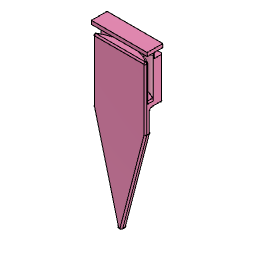
Fliegenfallenkleberfesthalter (Autodesk Fusion 360 design; units mm, degrees)
Autodesk Fusion 360 part; units mm, degrees
note: some values were not read from the file. Set by a fixed rule: which sketch regions a step uses.
sketch "Sketch1" plane through (0, 0, 0) normal (0, 0, 1) x (1, 0, 0)
  line L0 (0, 5) -> (15, 5)
  line L1 (15, 5) -> (15, 0)
  line L2 (15, 0) -> (0, 0)
  line L3 (0, 0) -> (0, 5)
  arc A0 (15, 0.75) -> (0, 0.75) centre (7.5, -11.5062) ccw
  arc A1 (15, 2.25) -> (0, 2.25) centre (7.5, -10.8125) ccw
  line L4 (0, 4.25) -> (15, 4.25) construction
  line L5 (0, 1.5) -> (15, 1.5)
  arc A2 (15, 2.5) -> (0, 2.5) centre (7.5, -10.5625) ccw
  dimension "d1" = 1.5
  dimension "d2" = 1.5
  dimension "d3" = 0.75
  dimension "d4" = 15
  dimension "d5" = 5
  dimension "d9" = 0.75
  dimension "d14" = 1.5
  dimension "d25" = 0.25
  dimension "d26" = 0.25
  constraint horizontal L0
  constraint vertical L1
  constraint horizontal L2
  constraint vertical L3
  constraint coincident L1 A0.start
  constraint coincident L3 A0.end
  constraint tangent A0 A1
  constraint coincident L1 A1.start
  constraint coincident L3 A1.end
  constraint coincident L2.end L3.start
  constraint horizontal A0.end A0.start
  constraint coincident L3 L4.start
  constraint coincident L1 L4.end
  constraint horizontal L4
  constraint tangent A1 L4
  constraint coincident L3 L5.start
  constraint coincident L1 L5.end
  constraint perpendicular L1 L5
  constraint coincident L1 A2.start
  constraint coincident L3 A2.end
  constraint equal A1 A2
  measures "d1" distance of A0.start A1.start
  measures "d2" distance of A0.end A1.end
  measures "d3" distance of L2.end A0.end
  measures "d4" distance of L1.end L2.end
  measures "d5" distance of L0.start L2.end
  measures "d9" distance of L0 L4
  measures "d14" distance of L2 L5
  measures "d25" distance of A1.start A2.start
  measures "d26" distance of A1.end A2.end
extrude "Extrude1" add sketch "Sketch1" against normal blind 2
extrude "Extrude2" add sketch "Sketch1" along normal blind 10 contours L0 L1 L3 A2 | L1 L3 A1 A2 | L1 L2 L3 A0 L5 | A0 L5
extrude "Extrude3" add sketch "Sketch1" against normal blind 35 contours L3 A0 L5 | L1 A0 L5 | L1 L2 L3 A0 L5
extrude "Extrude4" add sketch "Sketch1" along normal blind 12 and the other way blind -10 contours L1 L3 A1 A2
sketch "Sketch2" plane through (0, 0, 0) normal (0, -1, 0) x (1, 0, 0)
  line L0 (15, -35) -> (15, 10)
  line L1 (15, 10) -> (0, 10)
  line L2 (0, 10) -> (0, -35)
  line L3 (0, -35) -> (15, -35)
  line L4 (-0.5, 13) -> (15.5, 13)
  line L5 (15.5, 13) -> (15.5, 12)
  line L6 (15.5, 12) -> (-0.5, 12)
  line L7 (-0.5, 12) -> (-0.5, 13)
  dimension "d33" = 1
  constraint horizontal L4
  constraint vertical L5
  constraint horizontal L6
  constraint vertical L7
  measures "d33" distance of L4.start L6.end
extrude "Extrude5" add sketch "Sketch2" against normal blind 4.5 contours L4 L5 L6 L7
chamfer "Chamfer1" distance 7 distance2 27 1 edges at (15, 0.75, -35) measured on face at (5, 1, -35)
chamfer "Chamfer2" distance 7 distance2 27 1 edges at (0, 0.75, -35) measured on face at (2.6667, 1, -35)
fillet "Fillet2" radius 0.4 28 edges at (11.5, 1.5, -21.5) (7.5, 1.5, -35) (3.5, 1.5, -21.5) (3.5, 0, -21.5) (11.5, 0, -21.5) (7.5, 0, -35) (8, 0.75, -35) (7, 0.75, -35) (15, 3.25, -2) (15, 0, 1) (15, 0.75, -8) (15, 1.5, -5) (15, 5, 4) (7.5, 5, -2) (7.5, 1.5, -2) (0, 5, 4) (0, 3.25, -2) (0, 1.5, -5) (0, 0.75, -8) (0, 0, 1) (7.5, 2.8627, 10) (15, 0.375, 10) (0, 0.375, 10) (15, 0.75, 5) (15, 1.5, 0) (0, 0.75, 5) (0, 1.5, 0) (7.5, 0, 10)
equation "d1 = d2"
equation "d26 = d25"
